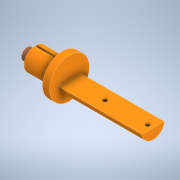
# Autodesk Inventor part: Eixo
Saved by Autodesk Inventor 2021 (Build 250183000, 183)
## iProperties
Created: 2021-04-08
Part Number: Eixo
Material: Genérico
Document SubType Name: Modeling
Designer: rubia
Density: 1 g/cm^3
Appearance: Laranja
Author: rubia
Autodesk Inventor part; units mm, degrees
ref_plane "YZ Plane" through (0, 0, 0) normal (1, 0, 0) x (0, 1, 0)
ref_plane "XZ Plane" through (0, 0, 0) normal (0, 1, 0) x (-1, 0, 0)
ref_plane "XY Plane" through (0, 0, 0) normal (0, 0, 1) x (1, 0, 0)
sketch "Esboço1" plane through (0, 0, 0) normal (0, 0, 1) x (1, 0, 0)
  line L0 (-30, 8) -> (28.9137, 8)
  line L1 (28.9137, 0) -> (28.9137, 8)
  line L2 (-30, 8) -> (-30, 14)
  line L3 (-30, 14) -> (-35, 14)
  line L4 (-35, 14) -> (-35, 8)
  line L5 (-35, 8) -> (-54, 8)
  line L6 (-54, 8) -> (-54, 4)
  line L7 (-54, 4) -> (-60, 4)
  line L8 (-60, 4) -> (-60, 0)
  line L9 (-60, 0) -> (28.9137, 0)
  point P0 (0, 0)
  dimension "d2" = 6
  dimension "d3" = 5
  dimension "d4" = 6
  dimension "d5" = 19
  dimension "d6" = 4
  dimension "d7" = 6
  constraints: 20 end point, 7 perpendicular, 1 horizontal
  measures "d2" distance of L0.start L2.end
  measures "d3" distance of L2.end L3.end
  measures "d4" distance of L3.end L4.end
  measures "d5" distance of L4.end L5.end
  measures "d6" distance of L5.end L6.end
  measures "d7" distance of L6.end L7.end
revolve "Revolução1" add sketch "Esboço1" angle 360 about axis through (-60, 0, 0) along (1, 0, 0)
sketch "Esboço2" plane through (0, 0, 0) normal (0, 1, 0) x (-1, 0, 0)
  line L0 (-28.9137, 8) -> (-28.9137, -8) projected
  line L1 (30, 8) -> (30, -8) projected
  line L2 (-28.9137, 8) -> (30, 8)
  line L3 (30, 8) -> (30, -8)
  line L4 (30, -8) -> (-28.9137, -8)
  line L5 (-28.9137, -8) -> (-28.9137, 8)
  point P0 (0, 0)
  constraints: 8 end point, 2 parallel, 1 horizontal, 1 perpendicular
extrude "Extrusão1" cut sketch "Esboço2" along normal blind 10 and the other way blind 1
sketch "Esboço3" plane through (0, -1, 0) normal (0, 1, 0) x (1, 0, 0)
  line L0 (-30, -14) -> (-30, 14) projected
  point P0 (0, 0)
  point P1 (-5, 0)
  point P2 (25, 0)
  dimension "d13" = 25
  dimension "d14" = 30
  measures "d13" distance from line of point (-5, 0) L0
  measures "d14" distance of point (-5, 0) point (25, 0)
hole "Furo1" at (-5, -1, 0) at (25, -1, 0) direction (0, -1, 0) diameter 3 end through all
thread "Rosca1" size "M8x0.75" class "6g" standard "ANSI Metric M Profile" length 7
fillet "Arredondamento1" radius 0.2 1 edges at (-60, -4, 0)
sketch "Esboço4" plane through (-54, 0, 0) normal (-1, 0, 0) x (0, 0, 1)
  circle A0 centre (0, 0) radius 8 projected
  line L0 (0, 8) -> (0.6, 8)
  line L1 (0.6, 8) -> (0.6, 6.6)
  line L2 (0.6, 6.6) -> (0, 6.6)
  line L3 (0, 6.6) -> (0, 8)
  line L4 (0, 8) -> (-0.6, 8)
  line L5 (-0.6, 8) -> (-0.6, 6.6)
  line L6 (-0.6, 6.6) -> (0, 6.6)
  line L7 (0, 6.6) -> (0, 8)
  point P0 (0.6, 7.9775)
  point P1 (-0.6, 7.9775)
  dimension "d25" = 0.6
  dimension "d26" = 1.4
  dimension "d27" = 0.6
  dimension "d28" = 1.4
  constraints: 16 end point, 4 parallel, 2 horizontal, 2 perpendicular, 2 other
  measures "d25" distance of L1.end L2.end
  measures "d26" distance of L0.end L1.end
  measures "d27" distance of L6.end L5.end
  measures "d28" distance of L5.end L4.end
extrude "Extrusão2" cut sketch "Esboço4" against normal blind 14 contours L1 L2 L3 A0 | A0 L3 L6 L5
